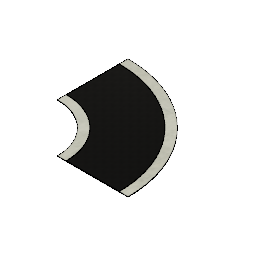
_Medium Turn - Ruby.ece09f05-70c2-46a3-bd11-477077b6546b (Autodesk Fusion 360 design; units mm, degrees)
Autodesk Fusion 360 part; units mm, degrees
sketch "Sketch1" plane through (0, 0, 0) normal (0, 0, 1) x (1, 0, 0)
  circle A0 centre (0, 0) radius 660.4
  circle A1 centre (0, 0) radius 1270
  line L0 (0, 0) -> (0, 1270)
  line L1 (0, 0) -> (1270, 0)
  dimension "d1" = 1320.8
  dimension "d2" = 609.6
  constraint coincident A0.centre A1.centre
  constraint coincident A1 L0.end
  constraint vertical L0
  constraint coincident A1 L1.end
  constraint perpendicular L0 L1
  measures "d1" diameter of A0
extrude "Extrude1" add sketch "Sketch1" along normal blind 6.35 contours A0 A1 L0 L1 picked at (60.2466, 1062.4911) makes body 1
sketch "Sketch2" plane through (0, 0, 6.35) normal (0, 0, 1) x (-1, 0, 0)
  line L0 (-660.4, 0) -> (-1270, 0)
  arc A0 (-1270, 0) -> (0, -1270) centre (0, 0) ccw
  line L1 (0, -1270) -> (0, -660.4)
  arc A1 (-660.4, 0) -> (0, -660.4) centre (0, 0) ccw
  arc A2 (-549.486, 101.6) -> (101.6, -549.486) centre (0, 0) ccw
  line L2 (101.6, -1367.8319) -> (101.6, -549.486)
  arc A3 (-1367.8319, 101.6) -> (101.6, -1367.8319) centre (0, 0) ccw
  line L3 (-549.486, 101.6) -> (-1367.8319, 101.6)
  line L4 (101.6, -549.486) -> (0, -549.486)
  line L5 (0, -549.486) -> (0, -1425.6301)
  line L6 (0, -1425.6301) -> (101.6, -1425.6301)
  line L7 (101.6, -1425.6301) -> (101.6, -549.486)
  line L8 (-549.486, 101.6) -> (-1530.0637, 101.6)
  line L9 (-1530.0637, 101.6) -> (-1530.0637, 0)
  line L10 (-1530.0637, 0) -> (-549.486, 0)
  line L11 (-549.486, 0) -> (-549.486, 101.6)
  dimension "d5" = 101.6
  dimension "d6" = 101.6
  dimension "d7" = 980.5776
  dimension "d8" = 101.6
  constraint horizontal L4
  constraint vertical L5
  constraint horizontal L6
  constraint vertical L7
  constraint horizontal L8
  constraint vertical L9
  constraint horizontal L10
  constraint vertical L11
  measures "d6" distance of A2.end L4.end
  measures "d7" distance of A2.start L8.end
  measures "d8" distance of A2.start L10.end
extrude "Extrude1'" add sketch "Sketch2" against normal blind 6.35 separate body contours A1 A2 L5 L10 | A0 A3 L5 L10 makes body 2 at (624.2927, 31.3282, 6.35) makes body 3 at (1310.251, 254.1211, 6.35) in component "90"
copy_body "CutPasteBodies1" bodies 1 removing the originals makes body 4 in component "90"
component "90" placed x (1, 0, 0) y (0, 1, 0) z (0, 0, 1) at (0, 0, 0)
